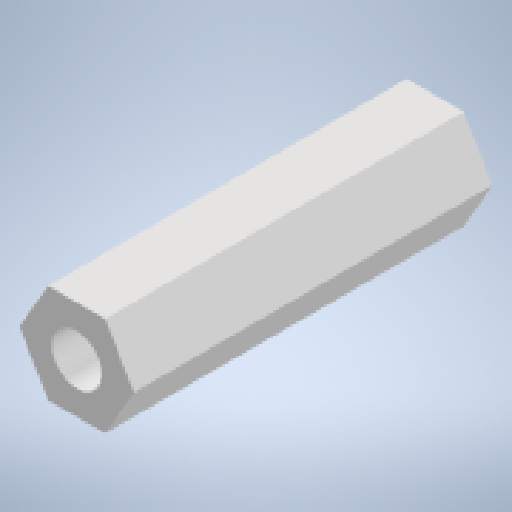
# Autodesk Inventor part: Montaje Manguera
Saved by Autodesk Inventor 2023.1 (Build 271208000, 208)
## iProperties
Created: 2022-11-04
Part Number: Montaje Manguera
Material: Generic
Document SubType Name: Modeling
Designer: Daniel Peña
Density: 1 g/cm^3
Appearance: Default
Author: Daniel Peña
Autodesk Inventor part; units mm, degrees
ref_plane "YZ Plane" through (0, 0, 0) normal (1, 0, 0) x (0, 1, 0)
ref_plane "XZ Plane" through (0, 0, 0) normal (0, 1, 0) x (-1, 0, 0)
ref_plane "XY Plane" through (0, 0, 0) normal (0, 0, 1) x (1, 0, 0)
sketch "Sketch1" plane through (0, 0, 0) normal (0, 0, 1) x (1, 0, 0)
  line L0 (7.9674, 0) -> (3.9837, -6.9)
  line L1 (3.9837, -6.9) -> (-3.9837, -6.9)
  line L2 (-3.9837, -6.9) -> (-7.9674, 0)
  line L3 (-7.9674, 0) -> (-3.9837, 6.9)
  line L4 (-3.9837, 6.9) -> (3.9837, 6.9)
  line L5 (3.9837, 6.9) -> (7.9674, 0)
  line L6 (3.4641, 0) -> (1.7321, -3)
  line L7 (1.7321, -3) -> (-1.7321, -3)
  line L8 (-1.7321, -3) -> (-3.4641, 0)
  line L9 (-3.4641, 0) -> (-1.7321, 3)
  line L10 (-1.7321, 3) -> (1.7321, 3)
  line L11 (1.7321, 3) -> (3.4641, 0)
  point P0 (0, 0)
  point P1 (0, 0)
  point P2 (0, 0)
  dimension "d0" = 13.8
  dimension "d1" = 6
  constraints: 24 end point, 2 coincident, 26 other
  measures "d0" distance between parallel lines of L1 L4
  measures "d1" distance between parallel lines of L7 L10
extrude "Extrusion1" add sketch "Sketch1" along normal blind 50
sketch "Sketch2" plane through (0, 0, 50) normal (0, 0, 1) x (1, 0, 0)
  line L0 (1.7321, -3) -> (-1.7321, -3) projected
  circle A0 centre (0, 0) radius 3.4641
  constraints: 1 coincident, 3 other
extrude "Extrusion2" cut sketch "Sketch2" against normal blind 50
body "Solid1"
